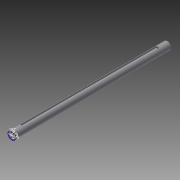
# Autodesk Inventor part: rod with key
Saved by Autodesk Inventor 2015 (Build 190159000, 159)
## iProperties
Created: 2015-01-20
Part Number: rod with key
Material: Generic
Document SubType Name: Modeling
Designer: mastkee16
Density: 1 g/cm^3
Appearance: Default
Author: mastkee16
Autodesk Inventor part; units mm, degrees
ref_plane "YZ Plane" through (0, 0, 0) normal (1, 0, 0) x (0, 1, 0)
ref_plane "XZ Plane" through (0, 0, 0) normal (0, 1, 0) x (-1, 0, 0)
ref_plane "XY Plane" through (0, 0, 0) normal (0, 0, 1) x (1, 0, 0)
sketch "Sketch1" plane through (0, 0, 0) normal (0, 0, 1) x (1, 0, 0)
  circle A0 centre (0, 0) radius 5.0254
  dimension "d0" = 10.0508
  constraints: 1 centre point, 1 coincident
  measures "d0" diameter of A0
extrude "Extrusion1" add sketch "Sketch1" along normal blind 202.8698
sketch "Sketch2" plane through (0, 0, 202.8698) normal (0, 0, 1) x (1, 0, 0)
  circle A0 centre (0, 0) radius 5.0254
  circle A1 centre (0, 0) radius 5.0254 projected
  line L0 (-1.9939, 4.6129) -> (1.9939, 4.6129)
  line L1 (1.9939, 4.6129) -> (1.9939, 2.619)
  line L2 (1.9939, 2.619) -> (-1.9939, 2.619)
  line L3 (-1.9939, 2.619) -> (-1.9939, 4.6129)
  arc A2 (1.9939, 4.6129) -> (-1.9939, 4.6129) centre (0, 0) ccw
  dimension "d3" = 3.9878
  dimension "d4" = 1.9939
  dimension "d5" = 1.9939
  constraints: 8 end point, 2 parallel, 2 point on circle, 1 centre point, 1 coincident, 1 horizontal, 1 perpendicular, 5 other
  measures "d3" distance between parallel lines of L1 L3
  measures "d4" distance of L0.end L1.end
  measures "d5" distance from line of point (0, 0) L3
extrude "Extrusion2" cut sketch "Sketch2" against normal blind 190.1698 contours L0 A0 | L1 L2 L3 L0
extrude "Extrusion3" add sketch "Sketch2" against normal blind 12.7 contours L0 A0 | L1 L2 L3 L0
body "Solid1"
